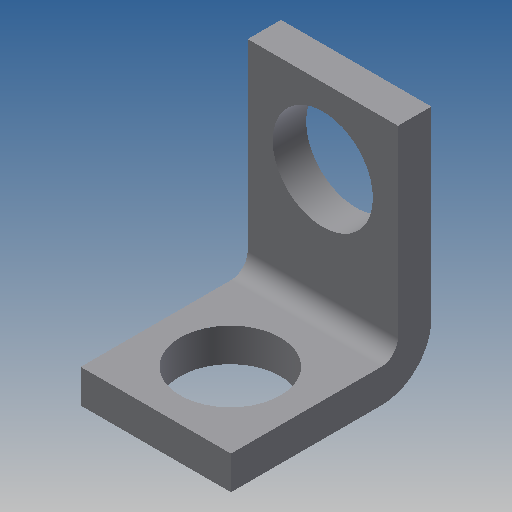
# Autodesk Inventor part: Pixy angle bracket
Saved by Autodesk Inventor 2017 (Build 210142000, 142)
## iProperties
Created: 2016-10-19
Part Number: Pixy angle bracket
Material: Generic
Document SubType Name: Modeling
Designer: James Yelland
Density: 1 g/cm^3
Appearance: Default
Author: James Yelland
Autodesk Inventor part; units mm, degrees
ref_plane "YZ Plane" through (0, 0, 0) normal (1, 0, 0) x (0, 1, 0)
ref_plane "XZ Plane" through (0, 0, 0) normal (0, 1, 0) x (-1, 0, 0)
ref_plane "XY Plane" through (0, 0, 0) normal (0, 0, 1) x (1, 0, 0)
sketch "Sketch1" plane through (0, 0, 0) normal (0, 1, 0) x (-1, 0, 0)
  line L0 (-1.9318, 2.5757) -> (2.5682, 2.5757)
  line L1 (2.5682, 2.5757) -> (2.5682, -3.4243)
  line L2 (2.5682, -3.4243) -> (-1.9318, -3.4243)
  line L3 (-1.9318, -3.4243) -> (-1.9318, 2.5757)
  line L4 (-1.9318, 2.5757) -> (2.5682, -3.4243) construction
  circle A0 centre (0.3372, 0.3257) radius 1.5
  point P0 (0, 0)
  dimension "d0" = 4.5
  dimension "d1" = 6
  dimension "d3" = 2.25
  constraints: 10 end point, 2 parallel, 1 centre point, 1 horizontal, 1 perpendicular, 1 point on line
  measures "d0" distance of L0.start L0.end
  measures "d1" distance of L0.end L1.end
  measures "d3" distance from line of L0 A0.centre
extrude "Extrusion1" add sketch "Sketch1" along normal blind 1
sketch "Sketch2" plane through (0, 1, 0) normal (0, 1, 0) x (1, 0, 0)
  circle A0 centre (-0.3372, -0.3257) radius 1.5 projected
  line L0 (-2.5682, -2.5757) -> (1.9318, -2.5757) projected
  line L1 (1.9318, -2.5757) -> (1.9318, 3.4243) projected
  line L2 (1.9318, 3.4243) -> (-2.5682, 3.4243) projected
  line L3 (-2.5682, 3.4243) -> (-2.5682, -2.5757) projected
  line L4 (-2.5682, 3.4243) -> (-2.5682, -2.5757) projected
  line L5 (-2.5682, 3.4243) -> (-2.5682, 2.4243)
  line L6 (-2.5682, 2.4243) -> (1.9318, 2.4243)
  line L7 (1.9318, 2.4243) -> (1.9318, 3.4243)
  line L8 (1.9318, 3.4243) -> (-2.5682, 3.4243)
  dimension "d6" = 1
  constraints: 8 end point, 2 parallel, 1 perpendicular, 1 point on line
  measures "d6" distance of L2.end L5.end
extrude "Extrusion2" add sketch "Sketch2" along normal blind 6 contours L3 L2 L1 L6
fillet "Fillet1" radius 1.5 1 edges at (-0.3182, 0, -3.4243)
sketch "Sketch3" plane through (1.9318, 7, -3.4243) normal (0, 0, -1) x (-1, 0, 0)
  line L0 (4.5, -5.5) -> (0, -5.5) projected
  line L1 (4.5, -5.5) -> (4.5, 0) projected
  line L2 (0, 0) -> (4.5, 0) projected
  line L3 (0, -5.5) -> (0, 0) projected
  line L4 (2.25, 0) -> (2.25, -2.25)
  circle A0 centre (2.25, -2.25) radius 1.5
  point P0 (1.9318, -7)
  dimension "d10" = 2.25
  dimension "d11" = 3
  constraints: 2 end point, 1 centre point, 1 coincident, 1 midpoint, 1 vertical
  measures "d10" distance of L4.start L4.end
  measures "d11" diameter of A0
extrude "Extrusion3" cut sketch "Sketch3" against normal blind 6 contours A0
fillet "Fillet2" radius 0.5 1 edges at (-0.3182, 1, -2.4243)
body "Solid1"
